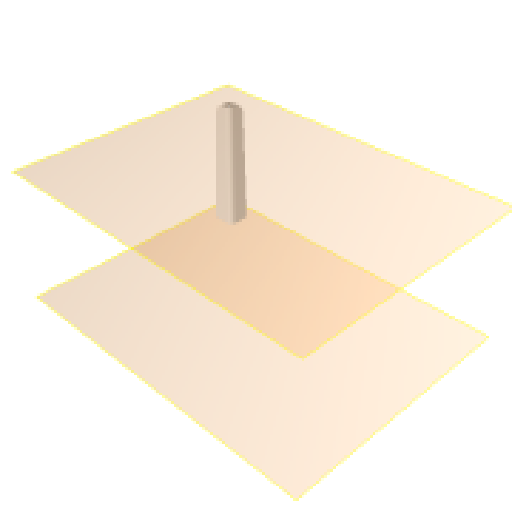
# Autodesk Inventor part: 60_Planktoscope_CornerPillars
Saved by Autodesk Inventor 2024.1 (Build 281209000, 209)
## iProperties
Created: 2024-08-10
Part Number: 60_Planktoscope_CornerPillars
Material: Generisch
Document SubType Name: Modeling
Designer: diederichbenedict
Density: 1 g/cm^3
Appearance: Vorgabe
Author: diederichbenedict
Autodesk Inventor part; units mm, degrees
ref_plane "YZ Plane" through (0, 0, 0) normal (1, 0, 0) x (0, 1, 0)
ref_plane "XZ Plane" through (0, 0, 0) normal (0, 1, 0) x (-1, 0, 0)
ref_plane "XY Plane" through (0, 0, 0) normal (0, 0, 1) x (1, 0, 0)
ref_plane "Arbeitsebene1" through (0, 0, 0) normal (0, 0, 1) x (1, 0, 0)
sketch "Skizze1" plane through (0, 0, 0) normal (0, 0, 1) x (1, 0, 0)
  line L0 (76.5043, -50) -> (76.5043, 50) projected
  arc A0 (96.5043, 50) -> (76.5043, 50) centre (86.5043, 50) ccw projected
  line L1 (96.5043, 50) -> (96.5043, -50) projected
  arc A1 (76.5043, -50) -> (96.5043, -50) centre (86.5043, -50) ccw projected
  line L2 (-95.8131, -50) -> (-95.8131, 50) projected
  arc A2 (-75.8131, 50) -> (-95.8131, 50) centre (-85.8131, 50) ccw projected
  line L3 (-75.8131, 50) -> (-75.8131, -50) projected
  arc A3 (-95.8131, -50) -> (-75.8131, -50) centre (-85.8131, -50) ccw projected
  line L4 (-118.5, -74.5) -> (-118.5, 74.5) projected
  arc A4 (-118.5, -74.5) -> (-103.5, -89.5) centre (-103.5, -74.5) ccw projected
  line L5 (56.1, -89.5) -> (-103.5, -89.5) projected
  line L6 (56.1, -83) -> (56.1, -89.5) projected
  arc A5 (71.1, -68) -> (56.1, -83) centre (71.1, -83) ccw projected
  line L7 (80.5, -68) -> (71.1, -68) projected
  arc A6 (95.5, -83) -> (80.5, -68) centre (80.5, -83) ccw projected
  line L8 (95.5, -89.5) -> (95.5, -83) projected
  line L9 (103.5, -89.5) -> (95.5, -89.5) projected
  arc A7 (103.5, -89.5) -> (118.5, -74.5) centre (103.5, -74.5) ccw projected
  line L10 (118.5, 74.5) -> (118.5, -74.5) projected
  arc A8 (118.5, 74.5) -> (103.5, 89.5) centre (103.5, 74.5) ccw projected
  line L11 (-103.5, 89.5) -> (103.5, 89.5) projected
  arc A9 (-103.5, 89.5) -> (-118.5, 74.5) centre (-103.5, 74.5) ccw projected
  circle A10 centre (-58.5, 18.7) radius 1.4 projected
  circle A11 centre (-58.5, 36.552) radius 1.4 projected
  circle A12 centre (57.5, 20.252) radius 1.4 projected
  circle A13 centre (57.5, 35) radius 1.4 projected
  circle A14 centre (-58.5, 8.7) radius 1.4 projected
  circle A15 centre (-58.5, -9.152) radius 1.4 projected
  circle A16 centre (57.5, 7.148) radius 1.4 projected
  circle A17 centre (57.5, -7.6) radius 1.4 projected
  circle A18 centre (103.5, 74.5) radius 1.4 projected
  circle A19 centre (103.5, -74.5) radius 1.4 projected
  circle A20 centre (-103.5, -74.5) radius 1.4 projected
  circle A21 centre (-103.5, 74.5) radius 1.4 projected
  line L12 (20.9567, 0.5738) -> (-20.9567, 0.5738) projected
  line L13 (-20.9567, 0.5738) -> (-20.9567, 30.6837) projected
  line L14 (-20.9567, 30.6837) -> (20.9567, 30.6837) projected
  line L15 (20.9567, 30.6837) -> (20.9567, 0.5738) projected
  circle A22 centre (73.1917, -22.4328) radius 1.4 projected
  circle A23 centre (43.1917, -22.4328) radius 1.4 projected
  circle A24 centre (13.1917, -22.4328) radius 1.4 projected
  circle A25 centre (-16.8083, -22.4328) radius 1.4 projected
  circle A26 centre (-46.8083, -22.4328) radius 1.4 projected
  circle A27 centre (-102.338, -1.3) radius 1.4 projected
  circle A28 centre (-102.338, 13.7) radius 1.4 projected
  circle A29 centre (-102.338, 28.7) radius 1.4 projected
  circle A30 centre (102.338, 28.7) radius 1.4 projected
  circle A31 centre (-73.1917, -22.4328) radius 1.4 projected
  circle A32 centre (-43.1917, -22.4328) radius 1.4 projected
  circle A33 centre (-13.1917, -22.4328) radius 1.4 projected
  circle A34 centre (16.8083, -22.4328) radius 1.4 projected
  circle A35 centre (46.8083, -22.4328) radius 1.4 projected
  circle A36 centre (102.338, -1.3) radius 1.4 projected
  circle A37 centre (102.338, 13.7) radius 1.4 projected
  circle A38 centre (-103.5, 74.5) radius 5
  line L16 (-116.5, 74.5) -> (-116.5, -74.5)
  arc A39 (-116.5, -74.5) -> (-103.5, -87.5) centre (-103.5, -74.5) ccw
  line L17 (-103.5, -87.5) -> (54.1, -87.5)
  line L18 (54.1, -87.5) -> (54.1, -83)
  arc A40 (71.1, -66) -> (54.1, -83) centre (71.1, -83) ccw
  line L19 (71.1, -66) -> (80.5, -66)
  arc A41 (97.5, -83) -> (80.5, -66) centre (80.5, -83) ccw
  line L20 (97.5, -83) -> (97.5, -87.5)
  line L21 (97.5, -87.5) -> (103.5, -87.5)
  arc A42 (103.5, -87.5) -> (116.5, -74.5) centre (103.5, -74.5) ccw
  line L22 (116.5, -74.5) -> (116.5, 74.5)
  arc A43 (116.5, 74.5) -> (103.5, 87.5) centre (103.5, 74.5) ccw
  line L23 (103.5, 87.5) -> (-103.5, 87.5)
  arc A44 (-103.5, 87.5) -> (-116.5, 74.5) centre (-103.5, 74.5) ccw
  line L24 (-98.5, 74.5) -> (-98.5, 87.5)
  line L25 (-103.5, 69.5) -> (-116.5, 69.5)
  circle A45 centre (-108.5, 79.5) radius 1.4 projected
  circle A46 centre (-108.5, -79.5) radius 1.4 projected
  circle A47 centre (108.5, 79.5) radius 1.4 projected
  circle A48 centre (108.5, -79.5) radius 1.4 projected
  point P0 (0, 0)
  dimension "d0" = 10
  dimension "d1" = 2
  constraints: 20 end point, 14 point on circle, 7 centre point, 2 perpendicular, 2 point on line, 1 coincident, 13 other
  measures "d0" diameter of A38
  measures "d1" radial gap between concentric circles of A9 A44
ref_plane "Arbeitsebene2" through (0, 0, 105.7) normal (0, 0, 1) x (1, 0, 0)
sketch "Skizze4" plane through (0, 0, 105.7) normal (0, 0, 1) x (1, 0, 0)
  line L0 (-98.5, 74.5) -> (-98.5, 87.5) projected
  circle A0 centre (-103.5, 74.5) radius 5 projected
  line L1 (-103.5, 69.5) -> (-116.5, 69.5) projected
  arc A1 (-103.5, 87.5) -> (-116.5, 74.5) centre (-103.5, 74.5) ccw projected
  arc A2 (-103.5, 83.5) -> (-112.5, 74.5) centre (-103.5, 74.5) ccw
  line L2 (-103.5, 83.5) -> (-98.5, 83.5)
  line L3 (-112.5, 74.5) -> (-112.5, 69.5)
  point P0 (0, 0)
  dimension "d8" = 4
  constraints: 4 end point, 2 point on circle, 2 point on line, 1 centre point, 1 horizontal, 1 perpendicular
  measures "d8" radial gap between concentric circles of A1 A2
loft "Erhebung1" add profiles "Skizze1", "Skizze4" contours A21 | A38 | A38 L25 L16 A44 L23 L24 | A45 / all
sketch "Skizze5" plane through (-103.5, 69.5, 0) normal (0, 0, -1) x (-1, 0, 0)
  circle A0 centre (0, 5) radius 3.25 projected
  circle A1 centre (0, 5) radius 1.4 projected
  circle A2 centre (5, 10) radius 1.4 projected
  point P0 (-103.5, -69.5)
extrude "Extrusion4" cut sketch "Skizze5" against normal blind 60 contours A1 | A2
fillet "Rundung1" radius 8 3 edges at (-109.864, 80.864, 105.7) (-101, 83.5, 105.7) (-112.5, 72, 105.7)
